Autodesk Inventor part; units mm, degrees
(part 2 of 2)
sketch "Sketch3" plane through (0, 0, -3) normal (0, 0, -1) x (-1, 0, 0)
  line L0 (5.881, -10.1787) -> (6.6726, -9.2707) projected
  line L1 (6.6726, -9.2707) -> (7.5242, -8.4183) projected
  line L2 (7.5242, -8.4183) -> (8.4301, -7.6298) projected
  line L3 (8.4301, -7.6298) -> (9.3899, -6.9034) projected
  line L4 (9.3899, -6.9034) -> (10.3924, -6.2477) projected
  line L5 (10.3924, -6.2477) -> (11.4408, -5.6607) projected
  line L6 (11.4408, -5.6607) -> (12.5232, -5.1482) projected
  line L7 (12.5232, -5.1482) -> (13.6379, -4.7115) projected
  line L8 (13.6379, -4.7115) -> (14.7806, -4.3515) projected
  line L9 (14.7806, -4.3515) -> (15.9403, -4.0716) projected
  line L10 (15.9403, -4.0716) -> (17.12, -3.8711) projected
  line L11 (17.12, -3.8711) -> (18.3057, -3.7515) projected
  line L12 (18.3057, -3.7515) -> (19.4988, -3.7135) projected
  line L13 (19.4988, -3.7135) -> (20.691, -3.7564) projected
  line L14 (20.691, -3.7564) -> (21.8743, -3.8803) projected
  line L15 (21.8743, -3.8803) -> (23.05, -4.0849) projected
  line L16 (23.05, -4.0849) -> (24.2044, -4.3678) projected
  line L17 (24.2044, -4.3678) -> (25.3402, -4.7298) projected
  line L18 (25.3402, -4.7298) -> (26.4473, -5.1673) projected
  line L19 (26.4473, -5.1673) -> (27.5214, -5.6792) projected
  line L20 (27.5214, -5.6792) -> (28.5612, -6.2641) projected
  line L21 (28.5612, -6.2641) -> (29.5556, -6.9168) projected
  line L22 (29.5556, -6.9168) -> (30.5076, -7.6388) projected
  line L23 (30.5076, -7.6388) -> (31.4066, -8.4225) projected
  line L24 (31.4066, -8.4225) -> (32.2527, -9.2695) projected
  line L25 (32.2527, -9.2695) -> (33.0399, -10.1719) projected
  line L26 (33.0399, -10.1719) -> (33.7574, -11.1167) projected
  line L27 (33.7574, -11.1167) -> (34.4081, -12.1076) projected
  line L28 (34.4081, -12.1076) -> (34.9897, -13.1403) projected
  line L29 (34.9897, -13.1403) -> (35.5038, -14.2179) projected
  line L30 (35.5038, -14.2179) -> (35.9446, -15.3298) projected
  line L31 (35.9446, -15.3298) -> (36.3075, -16.4694) projected
  line L32 (36.3075, -16.4694) -> (36.5936, -17.6366) projected
  line L33 (36.5936, -17.6366) -> (36.7981, -18.8157) projected
  line L34 (36.7981, -18.8157) -> (36.9211, -20.0072) projected
  line L35 (36.9211, -20.0072) -> (36.9632, -21.2132) projected
  line L36 (36.9632, -21.2132) -> (36.9221, -22.4103) projected
  line L37 (36.9221, -22.4103) -> (36.8004, -23.5952) projected
  line L38 (36.8004, -23.5952) -> (36.5978, -24.7695) projected
  line L39 (36.5978, -24.7695) -> (36.314, -25.9342) projected
  line L40 (36.314, -25.9342) -> (35.9529, -27.073) projected
  line L41 (35.9529, -27.073) -> (35.5136, -28.186) projected
  line L42 (35.5136, -28.186) -> (35.0001, -29.2661) projected
  line L43 (35.0001, -29.2661) -> (34.4181, -30.3023) projected
  line L44 (34.4181, -30.3023) -> (33.7658, -31.2978) projected
  line L45 (33.7658, -31.2978) -> (33.0454, -32.2477) projected
  line L46 (33.0454, -32.2477) -> (32.2538, -33.1556) projected
  line L47 (32.2538, -33.1556) -> (31.4021, -34.0081) projected
  line L48 (31.4021, -34.0081) -> (30.4963, -34.7966) projected
  line L49 (30.4963, -34.7966) -> (29.5366, -35.523) projected
  line L50 (29.5366, -35.523) -> (28.534, -36.1787) projected
  line L51 (28.534, -36.1787) -> (27.4856, -36.7657) projected
  line L52 (27.4856, -36.7657) -> (26.4032, -37.2782) projected
  line L53 (26.4032, -37.2782) -> (25.2885, -37.7149) projected
  line L54 (25.2885, -37.7149) -> (24.1458, -38.0749) projected
  line L55 (24.1458, -38.0749) -> (22.9861, -38.3548) projected
  line L56 (22.9861, -38.3548) -> (21.8064, -38.5553) projected
  line L57 (21.8064, -38.5553) -> (20.6207, -38.6749) projected
  line L58 (20.6207, -38.6749) -> (19.4276, -38.7129) projected
  line L59 (19.4276, -38.7129) -> (18.2354, -38.67) projected
  line L60 (18.2354, -38.67) -> (17.0521, -38.5461) projected
  line L61 (17.0521, -38.5461) -> (15.8764, -38.3415) projected
  line L62 (15.8764, -38.3415) -> (14.722, -38.0586) projected
  line L63 (14.722, -38.0586) -> (13.5862, -37.6966) projected
  line L64 (13.5862, -37.6966) -> (12.4791, -37.2591) projected
  line L65 (12.4791, -37.2591) -> (11.405, -36.7472) projected
  line L66 (11.405, -36.7472) -> (10.3652, -36.1622) projected
  line L67 (10.3652, -36.1622) -> (9.3708, -35.5096) projected
  line L68 (9.3708, -35.5096) -> (8.4188, -34.7876) projected
  line L69 (8.4188, -34.7876) -> (7.5197, -34.0039) projected
  line L70 (7.5197, -34.0039) -> (6.6737, -33.1569) projected
  line L71 (6.6737, -33.1569) -> (5.8865, -32.2545) projected
  line L72 (5.8865, -32.2545) -> (5.169, -31.3097) projected
  line L73 (5.169, -31.3097) -> (4.5183, -30.3188) projected
  line L74 (4.5183, -30.3188) -> (3.9367, -29.2861) projected
  line L75 (3.9367, -29.2861) -> (3.4226, -28.2085) projected
  line L76 (3.4226, -28.2085) -> (2.9818, -27.0966) projected
  line L77 (2.9818, -27.0966) -> (2.6189, -25.957) projected
  line L78 (2.6189, -25.957) -> (2.3328, -24.7898) projected
  line L79 (2.3328, -24.7898) -> (2.1283, -23.6107) projected
  line L80 (2.1283, -23.6107) -> (2.0053, -22.4191) projected
  line L81 (2.0053, -22.4191) -> (1.9632, -21.2132) projected
  line L82 (1.9632, -21.2132) -> (2.0043, -20.0161) projected
  line L83 (2.0043, -20.0161) -> (2.126, -18.8312) projected
  line L84 (2.126, -18.8312) -> (2.3286, -17.6568) projected
  line L85 (2.3286, -17.6568) -> (2.6124, -16.4922) projected
  line L86 (2.6124, -16.4922) -> (2.9734, -15.3534) projected
  line L87 (2.9734, -15.3534) -> (3.4128, -14.2404) projected
  line L88 (3.4128, -14.2404) -> (3.9263, -13.1603) projected
  line L89 (3.9263, -13.1603) -> (4.5083, -12.1241) projected
  line L90 (4.5083, -12.1241) -> (5.1606, -11.1286) projected
  line L91 (5.1606, -11.1286) -> (5.881, -10.1787) projected
  line L92 (37.0609, -39.3941) -> (37.1975, -39.2009) projected
  line L93 (37.1975, -39.2009) -> (37.3596, -39.0271) projected
  line L94 (37.3596, -39.0271) -> (37.5425, -38.878) projected
  line L95 (37.5425, -38.878) -> (37.7456, -38.7536) projected
  line L96 (37.7456, -38.7536) -> (37.9627, -38.6587) projected
  line L97 (37.9627, -38.6587) -> (38.1936, -38.593) projected
  line L98 (38.1936, -38.593) -> (38.4284, -38.5598) projected
  line L99 (38.4284, -38.5598) -> (38.6677, -38.5588) projected
  line L100 (38.6677, -38.5588) -> (38.9026, -38.5901) projected
  line L101 (38.9026, -38.5901) -> (39.1338, -38.6538) projected
  line L102 (39.1338, -38.6538) -> (39.3518, -38.7471) projected
  line L103 (39.3518, -38.7471) -> (39.5569, -38.8704) projected
  line L104 (39.5569, -38.8704) -> (39.742, -39.0192) projected
  line L105 (39.742, -39.0192) -> (39.9067, -39.1939) projected
  line L106 (39.9067, -39.1939) -> (40.0457, -39.3884) projected
  line L107 (40.0457, -39.3884) -> (40.1575, -39.6027) projected
  line L108 (40.1575, -39.6027) -> (40.2391, -39.8291) projected
  line L109 (40.2391, -39.8291) -> (40.2879, -40.0625) projected
  line L110 (40.2879, -40.0625) -> (40.3051, -40.3051) projected
  line L111 (40.3051, -40.3051) -> (40.2879, -40.547) projected
  line L112 (40.2879, -40.547) -> (40.2396, -40.7792) projected
  line L113 (40.2396, -40.7792) -> (40.1593, -41.0037) projected
  line L114 (40.1593, -41.0037) -> (40.0492, -41.216) projected
  line L115 (40.0492, -41.216) -> (39.9126, -41.4092) projected
  line L116 (39.9126, -41.4092) -> (39.7505, -41.5831) projected
  line L117 (39.7505, -41.5831) -> (39.5677, -41.7322) projected
  line L118 (39.5677, -41.7322) -> (39.3645, -41.8566) projected
  line L119 (39.3645, -41.8566) -> (39.1474, -41.9514) projected
  line L120 (39.1474, -41.9514) -> (38.9165, -42.0171) projected
  line L121 (38.9165, -42.0171) -> (38.6818, -42.0504) projected
  line L122 (38.6818, -42.0504) -> (38.4425, -42.0513) projected
  line L123 (38.4425, -42.0513) -> (38.2075, -42.0201) projected
  line L124 (38.2075, -42.0201) -> (37.9764, -41.9564) projected
  line L125 (37.9764, -41.9564) -> (37.7583, -41.8631) projected
  line L126 (37.7583, -41.8631) -> (37.5533, -41.7398) projected
  line L127 (37.5533, -41.7398) -> (37.3681, -41.5909) projected
  line L128 (37.3681, -41.5909) -> (37.2034, -41.4163) projected
  line L129 (37.2034, -41.4163) -> (37.0645, -41.2218) projected
  line L130 (37.0645, -41.2218) -> (36.9527, -41.0075) projected
  line L131 (36.9527, -41.0075) -> (36.8711, -40.7811) projected
  line L132 (36.8711, -40.7811) -> (36.8222, -40.5477) projected
  line L133 (36.8222, -40.5477) -> (36.8051, -40.3051) projected
  line L134 (36.8051, -40.3051) -> (36.8223, -40.0632) projected
  line L135 (36.8223, -40.0632) -> (36.8705, -39.831) projected
  line L136 (36.8705, -39.831) -> (36.9509, -39.6064) projected
  line L137 (36.9509, -39.6064) -> (37.0609, -39.3941) projected
  line L138 (-0.0172, -0.2419) -> (-0.0655, -0.4741) projected
  line L139 (-0.0655, -0.4741) -> (-0.1458, -0.6986) projected
  line L140 (-0.1458, -0.6986) -> (-0.2559, -0.9109) projected
  line L141 (-0.2559, -0.9109) -> (-0.3925, -1.1041) projected
  line L142 (-0.3925, -1.1041) -> (-0.5545, -1.278) projected
  line L143 (-0.5545, -1.278) -> (-0.7374, -1.4271) projected
  line L144 (-0.7374, -1.4271) -> (-0.9405, -1.5515) projected
  line L145 (-0.9405, -1.5515) -> (-1.1576, -1.6464) projected
  line L146 (-1.1576, -1.6464) -> (-1.3885, -1.7121) projected
  line L147 (-1.3885, -1.7121) -> (-1.6233, -1.7453) projected
  line L148 (-1.6233, -1.7453) -> (-1.8626, -1.7462) projected
  line L149 (-1.8626, -1.7462) -> (-2.0976, -1.715) projected
  line L150 (-2.0976, -1.715) -> (-2.3287, -1.6513) projected
  line L151 (-2.3287, -1.6513) -> (-2.5468, -1.558) projected
  line L152 (-2.5468, -1.558) -> (-2.7518, -1.4347) projected
  line L153 (-2.7518, -1.4347) -> (-2.9369, -1.2858) projected
  line L154 (-2.9369, -1.2858) -> (-3.1017, -1.1112) projected
  line L155 (-3.1017, -1.1112) -> (-3.2406, -0.9167) projected
  line L156 (-3.2406, -0.9167) -> (-3.3524, -0.7024) projected
  line L157 (-3.3524, -0.7024) -> (-3.434, -0.476) projected
  line L158 (-3.434, -0.476) -> (-3.4828, -0.2426) projected
  line L159 (-3.4828, -0.2426) -> (-3.5, 0) projected
  line L160 (-3.5, 0) -> (-3.4828, 0.2419) projected
  line L161 (-3.4828, 0.2419) -> (-3.4345, 0.4741) projected
  line L162 (-3.4345, 0.4741) -> (-3.3542, 0.6986) projected
  line L163 (-3.3542, 0.6986) -> (-3.2441, 0.911) projected
  line L164 (-3.2441, 0.911) -> (-3.1075, 1.1041) projected
  line L165 (-3.1075, 1.1041) -> (-2.9455, 1.278) projected
  line L166 (-2.9455, 1.278) -> (-2.7626, 1.4271) projected
  line L167 (-2.7626, 1.4271) -> (-2.5595, 1.5515) projected
  line L168 (-2.5595, 1.5515) -> (-2.3424, 1.6464) projected
  line L169 (-2.3424, 1.6464) -> (-2.1115, 1.7121) projected
  line L170 (-2.1115, 1.7121) -> (-1.8767, 1.7453) projected
  line L171 (-1.8767, 1.7453) -> (-1.6374, 1.7462) projected
  line L172 (-1.6374, 1.7462) -> (-1.4025, 1.715) projected
  line L173 (-1.4025, 1.715) -> (-1.1713, 1.6513) projected
  line L174 (-1.1713, 1.6513) -> (-0.9532, 1.558) projected
  line L175 (-0.9532, 1.558) -> (-0.7482, 1.4347) projected
  line L176 (-0.7482, 1.4347) -> (-0.5631, 1.2858) projected
  line L177 (-0.5631, 1.2858) -> (-0.3983, 1.1112) projected
  line L178 (-0.3983, 1.1112) -> (-0.2594, 0.9167) projected
  line L179 (-0.2594, 0.9167) -> (-0.1476, 0.7024) projected
  line L180 (-0.1476, 0.7024) -> (-0.066, 0.476) projected
  line L181 (-0.066, 0.476) -> (-0.0172, 0.2426) projected
  line L182 (-0.0172, 0.2426) -> (0, 0) projected
  line L183 (0, 0) -> (-0.0172, -0.2419) projected
  line L184 (39.5312, -46.3784) -> (40.1775, -46.0183) projected
  line L185 (40.1775, -46.0183) -> (40.7848, -45.6019) projected
  line L186 (40.7848, -45.6019) -> (41.3538, -45.1293) projected
  line L187 (41.3538, -45.1293) -> (41.8742, -44.6089) projected
  line L188 (41.8742, -44.6089) -> (42.3468, -44.0399) projected
  line L189 (42.3468, -44.0399) -> (42.7631, -43.4326) projected
  line L190 (42.7631, -43.4326) -> (43.1233, -42.7863) projected
  line L191 (43.1233, -42.7863) -> (43.4214, -42.1122) projected
  line L192 (43.4214, -42.1122) -> (43.6568, -41.4105) projected
  line L193 (43.6568, -41.4105) -> (43.8263, -40.6918) projected
  line L194 (43.8263, -40.6918) -> (43.9282, -39.962) projected
  line L195 (43.9282, -39.962) -> (43.9632, -39.2184) projected
  line L196 (43.9632, -39.2184) -> (43.9632, -21.2184) projected
  line L197 (43.9632, -21.2184) -> (43.9215, -19.7537) projected
  line L198 (43.9215, -19.7537) -> (43.7989, -18.3011) projected
  line L199 (43.7989, -18.3011) -> (43.5951, -16.8595) projected
  line L200 (43.5951, -16.8595) -> (43.3097, -15.4268) projected
  line L201 (43.3097, -15.4268) -> (42.9452, -14.0143) projected
  line L202 (42.9452, -14.0143) -> (42.5022, -12.626) projected
  line L203 (42.5022, -12.626) -> (41.9811, -11.2619) projected
  line L204 (41.9811, -11.2619) -> (41.3863, -9.9332) projected
  line L205 (41.3863, -9.9332) -> (40.7162, -8.6371) projected
  line L206 (40.7162, -8.6371) -> (39.9753, -7.3813) projected
  line L207 (39.9753, -7.3813) -> (39.1662, -6.1711) projected
  line L208 (39.1662, -6.1711) -> (38.2885, -5.0051) projected
  line L209 (38.2885, -5.0051) -> (37.3497, -3.8932) projected
  line L210 (37.3497, -3.8932) -> (36.3477, -2.8337) projected
  line L211 (36.3477, -2.8337) -> (35.2883, -1.8318) projected
  line L212 (35.2883, -1.8318) -> (34.1764, -0.893) projected
  line L213 (34.1764, -0.893) -> (33.0104, -0.0153) projected
  line L214 (33.0104, -0.0153) -> (31.8002, 0.7938) projected
  line L215 (31.8002, 0.7938) -> (30.5443, 1.5347) projected
  line L216 (30.5443, 1.5347) -> (29.2482, 2.2048) projected
  line L217 (29.2482, 2.2048) -> (27.9196, 2.7995) projected
  line L218 (27.9196, 2.7995) -> (26.5555, 3.3206) projected
  line L219 (26.5555, 3.3206) -> (25.1672, 3.7636) projected
  line L220 (25.1672, 3.7636) -> (23.7547, 4.1281) projected
  line L221 (23.7547, 4.1281) -> (22.322, 4.4136) projected
  line L222 (22.322, 4.4136) -> (20.8805, 4.6173) projected
  line L223 (20.8805, 4.6173) -> (19.4279, 4.7399) projected
  line L224 (19.4279, 4.7399) -> (17.9632, 4.7816) projected
  line L225 (17.9632, 4.7816) -> (-0.0368, 4.7816) projected
  line L226 (-0.0368, 4.7816) -> (-0.7805, 4.7466) projected
  line L227 (-0.7805, 4.7466) -> (-1.5103, 4.6447) projected
  line L228 (-1.5103, 4.6447) -> (-2.229, 4.4751) projected
  line L229 (-2.229, 4.4751) -> (-2.9307, 4.2397) projected
  line L230 (-2.9307, 4.2397) -> (-3.6048, 3.9416) projected
  line L231 (-3.6048, 3.9416) -> (-4.2511, 3.5814) projected
  line L232 (-4.2511, 3.5814) -> (-4.8584, 3.1651) projected
  line L233 (-4.8584, 3.1651) -> (-5.4274, 2.6925) projected
  line L234 (-5.4274, 2.6925) -> (-5.9478, 2.1721) projected
  line L235 (-5.9478, 2.1721) -> (-6.4204, 1.6031) projected
  line L236 (-6.4204, 1.6031) -> (-6.8367, 0.9958) projected
  line L237 (-6.8367, 0.9958) -> (-7.1969, 0.3495) projected
  line L238 (-7.1969, 0.3495) -> (-7.495, -0.3246) projected
  line L239 (-7.495, -0.3246) -> (-7.7304, -1.0263) projected
  line L240 (-7.7304, -1.0263) -> (-7.8999, -1.745) projected
  line L241 (-7.8999, -1.745) -> (-8.0018, -2.4748) projected
  line L242 (-8.0018, -2.4748) -> (-8.0368, -3.2184) projected
  line L243 (-8.0368, -3.2184) -> (-8.0368, -47.2184) projected
  line L244 (-8.0368, -47.2184) -> (35.9632, -47.2184) projected
  line L245 (35.9632, -47.2184) -> (36.7069, -47.1834) projected
  line L246 (36.7069, -47.1834) -> (37.4366, -47.0815) projected
  line L247 (37.4366, -47.0815) -> (38.1554, -46.9119) projected
  line L248 (38.1554, -46.9119) -> (38.8571, -46.6766) projected
  line L249 (38.8571, -46.6766) -> (39.5312, -46.3784) projected
extrude "Extrusion3" add sketch "Sketch3" along normal blind 1
body "Solid1"
